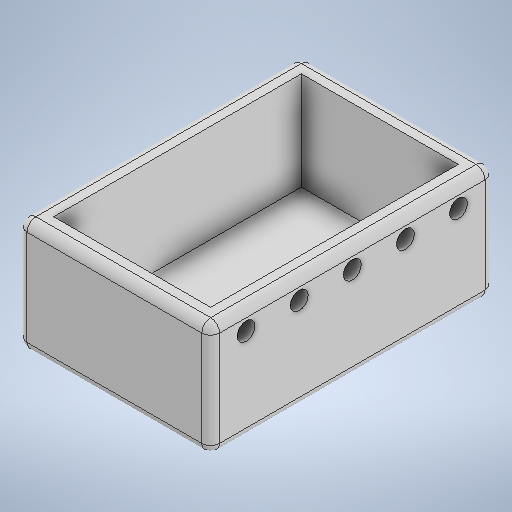
# Autodesk Inventor part: Part185
Saved by Autodesk Inventor 2025 (Build 290162000, 162)
## iProperties
Created: 2024-07-26
Part Number: Part185
Material: Generic
Document SubType Name: Modeling
Designer: Isaac
Density: 1 g/cm^3
Appearance: Default
Author: Isaac
Autodesk Inventor part; units mm, degrees
ref_plane "YZ Plane" through (0, 0, 0) normal (1, 0, 0) x (0, 1, 0)
ref_plane "XZ Plane" through (0, 0, 0) normal (0, 1, 0) x (-1, 0, 0)
ref_plane "XY Plane" through (0, 0, 0) normal (0, 0, 1) x (1, 0, 0)
sketch "Sketch1" plane through (0, 0, 0) normal (0, 0, 1) x (1, 0, 0)
  line L0 (-107.95, 63.5) -> (107.95, 63.5)
  line L1 (107.95, 63.5) -> (107.95, -63.5)
  line L2 (107.95, -63.5) -> (-107.95, -63.5)
  line L3 (-107.95, -63.5) -> (-107.95, 63.5)
  line L4 (-107.95, 63.5) -> (107.95, -63.5) construction
  line L5 (107.95, 63.5) -> (-107.95, -63.5) construction
  point P0 (0, 0)
  dimension "d0" = 215.9
  dimension "d1" = 127
  constraints: 12 end point, 2 midpoint, 2 parallel, 1 horizontal, 1 perpendicular
  measures "d0" distance of L0.start L0.end
  measures "d1" distance of L2.end L0.start
extrude "Extrusion1" add sketch "Sketch1" along normal blind 317.5
fillet "Fillet1" radius 10 12 edges at (0, 63.5, 317.5) (-107.95, 63.5, 158.75) (0, 63.5, 0) (107.95, 63.5, 158.75) (107.95, 0, 317.5) (107.95, -63.5, 158.75) (107.95, 0, 0) (0, -63.5, 317.5) (-107.95, 0, 317.5) (0, -63.5, 0) (-107.95, 0, 0) (-107.95, -63.5, 158.75)
sketch "Sketch4" plane through (-97.95, 63.5, 10) normal (0, 1, 0) x (1, 0, 0)
  line L0 (10, -10) -> (185.9, -10)
  line L1 (185.9, -10) -> (185.9, -287.5)
  line L2 (185.9, -287.5) -> (10, -287.5)
  line L3 (10, -287.5) -> (10, -10)
  line L4 (0, 0) -> (195.9, 0) projected
  line L5 (195.9, 0) -> (195.9, -297.5) projected
  line L6 (195.9, -297.5) -> (0, -297.5) projected
  line L7 (0, -297.5) -> (0, 0) projected
  point P0 (97.95, 10)
  point P1 (97.95, -10)
  dimension "d20" = 10
  dimension "d21" = 10
  dimension "d22" = 10
  dimension "d23" = 10
  constraints: 8 end point, 2 parallel, 1 horizontal, 1 midpoint, 1 perpendicular
  measures "d20" distance from line of L4 point (97.95, -10)
  measures "d21" distance between parallel lines of L5 L1
  measures "d22" distance between parallel lines of L6 L2
  measures "d23" distance between parallel lines of L7 L3
extrude "Extrusion4" cut sketch "Sketch4" against normal blind 110 contours L0 L1 L2 L3
sketch "Sketch5" plane through (107.95, -53.5, 10) normal (1, 0, 0) x (0, 0, -1)
  circle A0 centre (-267.75, 94.1117) radius 10
  circle A1 centre (-208.25, 94.1117) radius 10
  circle A2 centre (-148.75, 94.1117) radius 10
  circle A3 centre (-89.25, 94.1117) radius 10
  circle A4 centre (-29.75, 94.1117) radius 10
  line L0 (-297.5, 107) -> (-297.5, 0) projected
  point P0 (10, 53.5)
  dimension "d26" = 20
  dimension "d27" = 20
  dimension "d28" = 20
  dimension "d29" = 20
  dimension "d30" = 20
  dimension "d31" = 29.75
  dimension "d32" = 59.5
  dimension "d33" = 59.5
  dimension "d34" = 59.5
  dimension "d35" = 59.5
  constraints: 5 centre point
  measures "d26" diameter of A0
  measures "d27" diameter of A1
  measures "d28" diameter of A2
  measures "d29" diameter of A3
  measures "d30" diameter of A4
  measures "d31" distance from line of L0 A0.centre
  measures "d32" distance of A0.centre A1.centre
  measures "d33" distance of A1.centre A2.centre
  measures "d34" distance of A3.centre A2.centre
  measures "d35" distance of A4.centre A3.centre
extrude "Extrusion5" cut sketch "Sketch5" against normal blind 59.5
equation "\"d36\" = d33"
body "Solid1"
